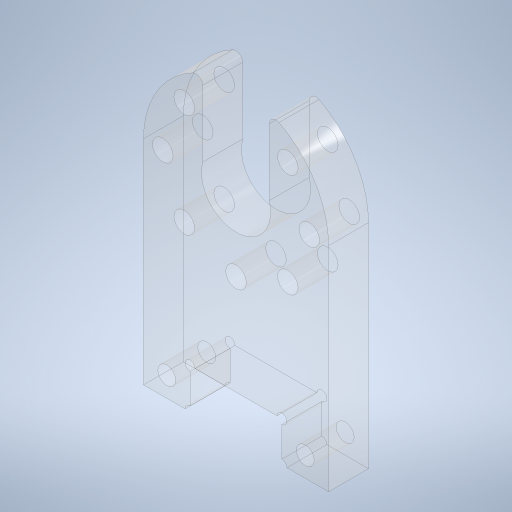
# Autodesk Inventor part: frame_knee_to_pelvis1
Saved by Autodesk Inventor 2024 (Build 280153000, 153)
## iProperties
Created: 2024-09-03
Part Number: frame_knee_to_pelvis1
Material: PMMA 플라스틱
Document SubType Name: Modeling
Designer: jmha0
Density: 1.188 g/cm^3
Appearance: 폴리카보네이트 - 선명
Mass: 6.14808 g
Surface Area: 33.2047 cm^2
Volume: 5.17515 cm^3
Author: jmha0
Autodesk Inventor part; units mm, degrees
ref_plane "YZ Plane" through (0, 0, 0) normal (1, 0, 0) x (0, 1, 0)
ref_plane "XZ Plane" through (0, 0, 0) normal (0, 1, 0) x (-1, 0, 0)
ref_plane "작업 평면1" through (0, 0, 0) normal (0, 0, 1) x (1, 0, 0)
sketch "스케치1" plane through (0, 0, 0) normal (0, 0, 1) x (1, 0, 0)
  circle A0 centre (-78.0165, 82.8266) radius 1.55
  circle A1 centre (-62.4602, 82.8266) radius 1.55
  circle A2 centre (-62.4602, 98.3829) radius 1.55
  circle A3 centre (-78.0165, 98.3829) radius 1.55
  circle A4 centre (-70.2383, 101.6047) radius 1.55
  circle A5 centre (-59.2383, 90.6047) radius 1.55
  circle A6 centre (-70.2383, 79.6047) radius 1.55
  circle A7 centre (-81.2383, 90.6047) radius 1.55
  arc A8 (-75.2383, 92.033) -> (-65.2383, 92.033) centre (-70.2383, 90.6047) ccw
  arc A9 (-75.2383, 103.5743) -> (-65.2383, 103.5743) centre (-70.2383, 90.6047) ccw
  line L0 (-65.2383, 95.8047) -> (-65.2383, 103.5743)
  line L1 (-75.2383, 95.8047) -> (-75.2383, 103.5743)
  line L2 (-65.2383, 95.8047) -> (-65.2383, 92.033)
  line L3 (-75.2383, 95.8047) -> (-75.2383, 92.033)
  circle A10 centre (-70.2383, 90.6047) radius 1.5
  circle A11 centre (-62.4602, 98.3829) radius 1.65
  circle A12 centre (-59.2383, 90.6047) radius 1.65
  circle A13 centre (-62.4602, 82.8266) radius 1.65
  circle A14 centre (-70.2383, 79.6047) radius 1.65
  circle A15 centre (-78.0165, 82.8266) radius 1.65
  circle A16 centre (-81.2383, 90.6047) radius 1.65
  circle A17 centre (-78.0165, 98.3829) radius 1.65
  line L4 (-56.3383, 90.6047) -> (-56.3383, 58.6047)
  line L5 (-84.1383, 90.6047) -> (-84.1383, 58.6047)
  arc A18 (-75.2383, 103.5743) -> (-84.1383, 90.6047) centre (-70.2383, 90.6047) ccw
  arc A19 (-56.3383, 90.6047) -> (-65.2383, 103.5743) centre (-70.2383, 90.6047) ccw
  line L6 (-84.1383, 58.6047) -> (-56.3383, 58.6047)
  arc A20 (-56.3383, 90.6047) -> (-65.2383, 103.5743) centre (-70.2383, 90.6047) ccw
  arc A21 (-75.2383, 103.5743) -> (-84.1383, 90.6047) centre (-70.2383, 90.6047) ccw
  point P0 (-52.7957, 62.4635)
  point P1 (-70.2383, 90.6047)
  point P2 (-85.25, 10.6344)
  point P3 (-75.25, 10.6344)
  point P4 (-94.15, -2.3352)
  point P5 (-66.35, -2.3352)
  point P6 (-88.3823, -54.5283)
  point P7 (-48.1823, -54.5283)
  point P8 (-88.3823, -54.5283)
  point P9 (-82.9823, -51.5283)
  point P10 (-53.5823, -51.5283)
  point P11 (-48.1823, -54.5283)
  point P12 (-84.1383, 90.6047)
  point P13 (-56.3383, 90.6047)
  dimension "d0" = 0.1
  dimension "d1" = 0.1
  dimension "d2" = 0.1
  dimension "d3" = 0.1
  dimension "d4" = 0.1
  dimension "d5" = 0.1
  dimension "d6" = 0.1
  dimension "d7" = 32
  dimension "d8" = 32
  dimension "d19" = 27.8
  constraints: 21 centre point, 14 end point, 10 point on circle, 7 vertical, 4 tangent, 1 coincident, 4 other
  measures "d0" radial gap between concentric circles of A2 A11
  measures "d1" radial gap between concentric circles of A5 A12
  measures "d2" radial gap between concentric circles of A1 A13
  measures "d3" radial gap between concentric circles of A6 A14
  measures "d4" radial gap between concentric circles of A0 A15
  measures "d5" radial gap between concentric circles of A7 A16
  measures "d6" radial gap between concentric circles of A3 A17
  measures "d7" distance of L4.start L4.end
  measures "d8" distance of L5.start L5.end
  measures "d19" distance between parallel lines of L4 L5
extrude "돌출1" add sketch "스케치1" along normal blind 6 contours A8 L2 L0 A9 L1 L3 | A9 L4 L6 L5 | A11 | A12 | A13 | A14 | A15 | A16 | A17
sketch "스케치2" plane through (0, 0, 6) normal (0, 0, 1) x (1, 0, 0)
  line L0 (-65.2383, 103.5743) -> (-65.2383, 92.033) projected
  arc A0 (-75.2383, 92.033) -> (-65.2383, 92.033) centre (-70.2383, 90.6047) ccw projected
  line L1 (-75.2383, 92.033) -> (-75.2383, 103.5743) projected
  arc A1 (-75.2383, 103.5743) -> (-84.1383, 90.6047) centre (-70.2383, 90.6047) ccw projected
  line L2 (-84.1383, 90.6047) -> (-84.1383, 58.6047) projected
  line L3 (-84.1383, 58.6047) -> (-56.3383, 58.6047) projected
  line L4 (-56.3383, 58.6047) -> (-56.3383, 90.6047) projected
  arc A2 (-56.3383, 90.6047) -> (-65.2383, 103.5743) centre (-70.2383, 90.6047) ccw projected
  line L5 (-84.1383, 58.6047) -> (-56.3383, 58.6047)
  line L6 (-56.3383, 58.6047) -> (-56.3383, 64.6047)
  line L7 (-56.3383, 64.6047) -> (-84.1383, 64.6047)
  line L8 (-84.1383, 64.6047) -> (-84.1383, 58.6047)
  line L9 (-84.1383, 58.6047) -> (-77.1383, 58.6047)
  line L10 (-77.1383, 58.6047) -> (-63.3383, 58.6047)
  line L11 (-63.3383, 58.6047) -> (-56.3383, 58.6047)
  line L12 (-63.3383, 58.6047) -> (-63.3383, 64.6047)
  line L13 (-77.1383, 58.6047) -> (-77.1383, 64.6047)
  point P0 (0, 0)
  point P1 (-56.3383, 61.6047)
  point P2 (-63.3383, 61.6047)
  dimension "d20" = 6
  dimension "d21" = 7
  dimension "d22" = 13.8
  dimension "d23" = 7
  constraints: 18 end point, 5 point on line, 3 perpendicular, 2 midpoint, 2 parallel, 1 collinear, 1 horizontal
  measures "d20" distance of L6.end L5.end
  measures "d21" distance of L2.end L9.end
  measures "d22" distance of L9.end L10.end
  measures "d23" distance of point (-56.338, 61.605) point (-63.338, 61.605)
extrude "돌출2" cut sketch "스케치2" against normal blind 10 contours L12 L3 L13 L7
sketch "스케치3" plane through (0, 0, 6) normal (0, 0, 1) x (1, 0, 0)
  line L0 (-63.3383, 64.6047) -> (-63.3383, 58.6047) projected
  line L1 (-63.3383, 58.6047) -> (-56.3383, 58.6047) projected
  line L2 (-56.3383, 58.6047) -> (-56.3383, 90.6047) projected
  arc A0 (-56.3383, 90.6047) -> (-65.2383, 103.5743) centre (-70.2383, 90.6047) ccw projected
  line L3 (-65.2383, 103.5743) -> (-65.2383, 92.033) projected
  arc A1 (-75.2383, 92.033) -> (-65.2383, 92.033) centre (-70.2383, 90.6047) ccw projected
  line L4 (-75.2383, 92.033) -> (-75.2383, 103.5743) projected
  arc A2 (-75.2383, 103.5743) -> (-84.1383, 90.6047) centre (-70.2383, 90.6047) ccw projected
  line L5 (-84.1383, 90.6047) -> (-84.1383, 58.6047) projected
  line L6 (-84.1383, 58.6047) -> (-77.1383, 58.6047) projected
  line L7 (-77.1383, 58.6047) -> (-77.1383, 64.6047) projected
  line L8 (-77.1383, 64.6047) -> (-63.3383, 64.6047) projected
  circle A3 centre (-59.8383, 61.6047) radius 1.35
  circle A4 centre (-80.6383, 61.6047) radius 1.35
  point P0 (0, 0)
  dimension "d26" = 2.7
  dimension "d27" = 2.7
  dimension "d30" = 20.8
  constraints: 2 centre point
  measures "d26" diameter of A3
  measures "d27" diameter of A4
  measures "d30" distance of A3.centre A4.centre
extrude "돌출3" cut sketch "스케치3" against normal blind 10 contours A3 | A4
fillet "모깎기1" radius 1 2 edges at (-75.2383, 103.5743, 3) (-65.2383, 103.5743, 3)
sketch "스케치5" plane through (0, 0, 6) normal (0, 0, 1) x (1, 0, 0)
  arc A0 (-63.7732, 102.9097) -> (-65.2383, 102.0245) centre (-64.2383, 102.0245) ccw projected
  line L0 (-65.2383, 102.0245) -> (-65.2383, 92.033) projected
  arc A1 (-75.2383, 92.033) -> (-65.2383, 92.033) centre (-70.2383, 90.6047) ccw projected
  line L1 (-75.2383, 92.033) -> (-75.2383, 102.0245) projected
  arc A2 (-75.2383, 102.0245) -> (-76.7034, 102.9097) centre (-76.2383, 102.0245) ccw projected
  arc A3 (-76.7034, 102.9097) -> (-84.1383, 90.6047) centre (-70.2383, 90.6047) ccw projected
  line L2 (-84.1383, 90.6047) -> (-84.1383, 58.6047) projected
  line L3 (-84.1383, 58.6047) -> (-77.1383, 58.6047) projected
  line L4 (-77.1383, 58.6047) -> (-77.1383, 64.6047) projected
  line L5 (-77.1383, 64.6047) -> (-63.3383, 64.6047) projected
  line L6 (-63.3383, 64.6047) -> (-63.3383, 58.6047) projected
  line L7 (-63.3383, 58.6047) -> (-56.3383, 58.6047) projected
  line L8 (-56.3383, 58.6047) -> (-56.3383, 90.6047) projected
  arc A4 (-56.3383, 90.6047) -> (-63.7732, 102.9097) centre (-70.2383, 90.6047) ccw projected
  circle A5 centre (-59.8383, 61.6047) radius 1.35 projected
  circle A6 centre (-80.6383, 61.6047) radius 1.35 projected
  circle A7 centre (-62.4602, 98.3829) radius 1.55 projected
  circle A8 centre (-59.2383, 90.6047) radius 1.55 projected
  circle A9 centre (-62.4602, 82.8266) radius 1.55 projected
  circle A10 centre (-70.2383, 79.6047) radius 1.55 projected
  circle A11 centre (-78.0165, 82.8266) radius 1.55 projected
  circle A12 centre (-81.2383, 90.6047) radius 1.55 projected
  circle A13 centre (-78.0165, 98.3829) radius 1.55 projected
  circle A14 centre (-77.1383, 58.6047) radius 0.75
  line L9 (-77.1383, 58.6047) -> (-77.1383, 64.6047) projected
  circle A15 centre (-77.1383, 64.6047) radius 0.75
  circle A16 centre (-63.3383, 64.6047) radius 0.75
  circle A17 centre (-63.3383, 58.6047) radius 0.75
  point P0 (0, 0)
  point P1 (-77.1383, 59.3547)
  point P2 (-77.8883, 58.6047)
  dimension "d32" = 1.5
  dimension "d33" = 1.5
  dimension "d34" = 1.5
  dimension "d35" = 1.5
  constraints: 4 centre point, 4 coincident
  measures "d32" diameter of A14
  measures "d33" diameter of A15
  measures "d34" diameter of A16
  measures "d35" diameter of A17
extrude "돌출4" cut sketch "스케치5" against normal blind 10 contours A17 L6 L7 | L7 L6 A17 | A16 L5 L6 | L6 L5 A16 | A15 L4 L5 | L5 L4 A15 | A14 L4 L3 picked at (-77.3024, 59.0737)
